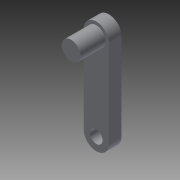
# Autodesk Inventor part: Geneva Frame
Saved by Autodesk Inventor 2018 (Build 220112000, 112)
## iProperties
Created: 2018-01-19
Part Number: Geneva Frame
Material: Generic
Document SubType Name: Modeling
Designer: Rus
Density: 1 g/cm^3
Appearance: Default
Author: Rus
Autodesk Inventor part; units mm, degrees
ref_plane "YZ Plane" through (0, 0, 0) normal (1, 0, 0) x (0, 1, 0)
ref_plane "XZ Plane" through (0, 0, 0) normal (0, 1, 0) x (-1, 0, 0)
ref_plane "XY Plane" through (0, 0, 0) normal (0, 0, 1) x (1, 0, 0)
sketch "Sketch1" plane through (0, 0, 0) normal (0, 0, 1) x (1, 0, 0)
  circle A0 centre (-124.6002, 78.2127) radius 9.525
  point P0 (0, 0)
  dimension "d0" = 19.05
  constraints: 1 centre point
  measures "d0" diameter of A0
extrude "Extrusion1" add sketch "Sketch1" along normal blind 16.9333
sketch "Sketch2" plane through (-124.6002, 78.2127, 0) normal (0, 0, -1) x (-1, 0, 0)
  circle A0 centre (0, 0) radius 9.525 projected
  line L0 (0, 0) -> (0, -87.9881) construction
  line L1 (-12.7, 0) -> (-12.7, -87.9881)
  line L2 (12.7, -87.9881) -> (12.7, 0)
  arc A1 (12.7, 0) -> (-12.7, 0) centre (0, 0) ccw
  arc A2 (-12.7, -87.9881) -> (12.7, -87.9881) centre (0, -87.9881) ccw
  line L3 (0, 0) -> (87.9881, 0) construction
  circle A3 centre (0, -87.9881) radius 6.35
  point P0 (-124.6002, -78.2127)
  point P1 (0, -43.9941)
  dimension "d6" = 87.9881
  dimension "d7" = 90
  dimension "d8" = 25.4
  dimension "d9" = 12.7
  constraints: 10 end point, 4 point on circle, 4 tangent, 3 centre point, 1 coincident, 1 horizontal, 1 midpoint, 1 parallel, 1 perpendicular, 1 vertical
  measures "d6" distance of L0.start L0.end
  measures "d7" angle of L0 L3
  measures "d8" diameter of A2
  measures "d9" diameter of A3
extrude "Extrusion2" add sketch "Sketch2" along normal blind 12.7 contours A0 | A1 L2 A2 L1
sketch "Sketch3" plane through (-124.6002, 78.2127, 16.9333) normal (0, 0, 1) x (1, 0, 0)
  circle A0 centre (0, 0) radius 9.525 projected
  point P0 (124.6002, -78.2127)
extrude "Extrusion3" add sketch "Sketch3" along normal blind 8.4667
body "Solid1"
